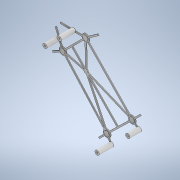
# Autodesk Inventor part: Grundform_Boden
Saved by Autodesk Inventor 2020.2 (Build 242310000, 310)
## iProperties
Created: 2020-03-04
Part Number: Grundform_Boden
Material: Generic
Document SubType Name: Modeling
Designer: Mara
Density: 1 g/cm^3
Appearance: Default
Author: Mara
Autodesk Inventor part; units mm, degrees
ref_plane "YZ Plane" through (0, 0, 0) normal (1, 0, 0) x (0, 1, 0)
ref_plane "XZ Plane" through (0, 0, 0) normal (0, 1, 0) x (-1, 0, 0)
ref_plane "XY Plane" through (0, 0, 0) normal (0, 0, 1) x (1, 0, 0)
sketch "Sketch1" plane through (0, 0, 0) normal (0, 0, 1) x (1, 0, 0)
  line L0 (-49.2977, 34.5359) -> (-22.38, 61.3045)
  line L1 (-47.8874, 33.1177) -> (-20.9698, 59.8864)
  line L2 (-49.2977, 34.5359) -> (-47.8874, 33.1177) construction
  circle A0 centre (-52.4729, 29.968) radius 5.563
  circle A1 centre (-52.4729, 29.968) radius 3.9984
  circle A2 centre (-17.7815, 64.4351) radius 5.563
  circle A3 centre (-17.7815, 64.4351) radius 3.9984
  line L3 (-13.9364, 68.4553) -> (0.7038, 78.9274)
  line L4 (-12.7631, 66.8356) -> (1.8771, 77.3077)
  line L5 (-57.711, 28.0946) -> (-68.2683, 22.3899)
  line L6 (-56.7093, 26.3625) -> (-67.2666, 20.6578)
  line L7 (-49.5894, 25.2106) -> (10.1162, -41.4966)
  circle A4 centre (14.4958, -44.9268) radius 5.563
  circle A5 centre (14.4958, -44.9268) radius 3.9984
  circle A6 centre (52.6405, -7.8239) radius 3.9984
  circle A7 centre (52.6405, -7.8239) radius 5.563
  line L8 (-48.0932, 26.5378) -> (11.6124, -40.1694)
  line L9 (-14.6001, 59.8716) -> (48.0505, -4.6808)
  line L10 (-13.1915, 61.292) -> (49.4591, -3.2604)
  line L11 (49.4227, -12.3618) -> (19.1106, -41.8201)
  line L12 (48.0258, -10.9306) -> (17.7136, -40.3888)
  line L13 (11.2885, -49.4721) -> (3.1929, -57.3557)
  line L14 (9.8883, -48.0441) -> (1.7927, -55.9277)
  line L15 (57.2511, -4.7111) -> (65.8331, 3.6764)
  line L16 (55.8523, -3.2817) -> (64.4343, 5.1058)
  line L17 (-39.0119, 41.9442) -> (29.6903, -28.7495)
  line L18 (-37.5936, 43.3546) -> (31.1246, -27.3556)
  line L19 (-55.5021, 34.6339) -> (-63.8979, 55.9393)
  line L20 (-53.6558, 35.4038) -> (-62.0516, 56.7092)
  line L21 (-23.223, 65.5915) -> (-56.073, 66.1322)
  line L22 (-23.2803, 63.5921) -> (-56.1303, 64.1329)
  circle A8 centre (-17.2221, 20.9576) radius 3.1804
  line L23 (13.0651, -39.5509) -> (-14.9644, 18.7175)
  line L24 (11.2563, -40.4044) -> (-16.7485, 17.8127)
  line L25 (-14.0533, 20.686) -> (47.9022, -4.9092)
  line L26 (-14.8421, 18.848) -> (47.1775, -6.7738)
  line L27 (-18.703, 58.9489) -> (-18.2564, 23.9652)
  line L28 (-16.7032, 58.9776) -> (-16.2565, 23.9879)
  line L29 (-47.4654, 27.5447) -> (-20.389, 20.6653)
  line L30 (-46.932, 29.4728) -> (-19.9371, 22.614)
  line L31 (0.7038, 78.9274) -> (1.8771, 77.3077)
  line L32 (-56.073, 66.1322) -> (-56.1303, 64.1329)
  line L33 (-62.0516, 56.7092) -> (-63.8979, 55.9393)
  line L34 (-68.2683, 22.3899) -> (-67.2666, 20.6578)
  line L35 (3.1929, -57.3557) -> (1.7927, -55.9277)
  line L36 (65.8331, 3.6764) -> (64.4343, 5.1058)
  point P0 (0, 0)
  point P1 (9.143, -43.4122)
  point P2 (-19.963, 60.8956)
  point P3 (18.6755, -41.2556)
  point P4 (19.8991, -43.603)
  point P5 (47.2964, -9.3692)
  point P6 (58.0343, -9.1855)
  point P7 (55.8444, -3.2761)
  point P8 (16.2732, -50.1982)
  point P9 (18.0227, -49.2289)
  point P10 (56.2951, -12.0181)
  point P11 (57.5423, -10.4544)
  point P12 (-20.321, 22.7115)
  point P13 (-20.9757, 59.8805)
  point P14 (-18.6091, 23.8197)
  point P15 (10.5981, -39.0362)
  point P16 (31.0842, -30.1838)
  point P17 (32.5185, -28.7899)
  point P18 (31.1246, -27.3556)
  point P19 (-13.0632, 18.1131)
  point P20 (-13.5186, 15.7119)
  point P21 (29.6903, -28.7495)
  point P22 (-20.0433, 22.4258)
  dimension "d49" = 6.3609
  dimension "d0" = 2
  dimension "d2" = 1
  dimension "d3" = 5.563
  dimension "d4" = 1.5646
  dimension "d6" = 1.5646
  dimension "d8" = 5.563
  dimension "d9" = 2
  dimension "d10" = 170.735
  dimension "d11" = 2
  dimension "d12" = 163.544
  dimension "d13" = 1.5646
  dimension "d17" = 7.9968
  dimension "d18" = 1.5646
  dimension "d19" = 7.9968
  dimension "d21" = 60.4275
  dimension "d22" = 66.8436
  dimension "d24" = 47.2075
  dimension "d25" = 2
  dimension "d26" = 2
  dimension "d27" = 81.433
  dimension "d28" = 93.011
  dimension "d29" = 53.2188
  dimension "d30" = 2
  dimension "d31" = 2
  dimension "d32" = 2
  dimension "d33" = 2
  dimension "d34" = 2
  dimension "d35" = 2
  dimension "d36" = 66.667
  dimension "d37" = 45.784
  dimension "d39" = 92.41
  dimension "d40" = 87.648
  dimension "d42" = 89.8
  dimension "d45" = 1
  dimension "d46" = 18
  dimension "d48" = 2
  dimension "d50" = 53.2132
  dimension "d51" = 27.126
  dimension "d52" = 44.9268
  dimension "d53" = 48.9027
  dimension "d54" = 29.968
  dimension "d55" = 20.9576
  dimension "d56" = 2
  dimension "d57" = 2
  dimension "d58" = 2
  dimension "d59" = 64.6596
  dimension "d60" = 67.0343
  dimension "d61" = 34.9897
  dimension "d62" = 27.8525
  dimension "d63" = 22.9
  dimension "d64" = 12
  dimension "d65" = 32.85
  dimension "d66" = 18
  dimension "d67" = 12
  dimension "d70" = 11.3
  dimension "d71" = 3.8451
  dimension "d72" = 5.4415
  dimension "d73" = 5.4358
  dimension "d74" = 5.2381
  dimension "d75" = 5.5409
  dimension "d76" = 5.4575
  dimension "d77" = 3.1128
  dimension "d78" = 2.6305
  dimension "d79" = 4.3021
  constraints: 75 end point, 25 parallel, 4 centre point, 4 coincident, 4 point on line, 2 perpendicular, 62 other
  measures "d0" distance between parallel lines of L1 L0
  measures "d2" distance from line of L0 point (-52.473, 29.968)
  measures "d3" distance of L0.start point (-52.473, 29.968)
  measures "d8" distance of L0.end point (-17.782, 64.435)
  measures "d9" distance between parallel lines of L4 L3
  measures "d10" angle of L3 L0
  measures "d11" distance between parallel lines of L6 L5
  measures "d12" angle of L1 L6
  measures "d17" diameter of A5
  measures "d19" diameter of A6
  measures "d21" distance of point (-52.473, 29.968) point (0, 0)
  measures "d22" distance of point (0, 0) point (-17.782, 64.435)
  measures "d24" distance of point (0, 0) point (14.496, -44.927)
  measures "d25" distance between parallel lines of L7 L8
  measures "d26" distance between parallel lines of L9 L10
  measures "d27" angle of L10 L4
  measures "d28" angle of L8 L1
  measures "d29" distance of point (0, 0) point (52.641, -7.824)
  measures "d30" distance between parallel lines of L11 L12
  measures "d31" distance between parallel lines of L13 L14
  measures "d32" distance between parallel lines of L15 L16
  measures "d33" distance between parallel lines of L18 L17
  measures "d34" distance between parallel lines of L20 L19
  measures "d35" distance between parallel lines of L21 L22
  measures "d36" angle of L0 L20
  measures "d37" angle of L0 L22
  measures "d39" angle of L14 L7
  measures "d40" angle of L12 L8
  measures "d42" angle of L10 L16
  measures "d45" distance from line of point (-17.222, 20.958) L18
  measures "d46" distance from line of L17 point (-52.473, 29.968)
  measures "d48" distance between parallel lines of L23 L24
  measures "d50" distance of point (52.641, -7.824) A5.centre
  measures "d51" distance of point (0, 0) point (-17.222, 20.958)
  measures "d52" vertical distance of point (0, 0) point (14.496, -44.927)
  measures "d53" distance of point (-52.473, 29.968) point (-17.782, 64.435)
  measures "d54" vertical distance of point (0, 0) point (-52.473, 29.968)
  measures "d55" vertical distance of point (-17.222, 20.958) point (0, 0)
  measures "d56" distance between parallel lines of L26 L25
  measures "d57" distance between parallel lines of L28 L27
  measures "d58" distance between parallel lines of L29 L30
  measures "d59" distance of L23.start L23.end
  measures "d60" distance of L25.start L25.end
  measures "d61" vertical distance of L28.start L28.end
  measures "d62" distance of L30.start L30.end
  measures "d63" distance of L20.start L20.end
  measures "d64" distance of L5.start L5.end
  measures "d65" horizontal distance of L22.start L22.end
  measures "d66" distance of L3.start L3.end
  measures "d67" distance of L15.start L15.end
  measures "d70" distance of L13.start L13.end
  measures "d71" horizontal distance of L3.start point (-17.782, 64.435)
  measures "d72" horizontal distance of point (-17.782, 64.435) L21.start
  measures "d73" vertical distance of point (-52.473, 29.968) L20.start
  measures "d74" horizontal distance of L5.start A1.centre
  measures "d75" horizontal distance of point (-52.473, 29.968) L30.start
  measures "d76" vertical distance of point (-17.782, 64.435) L28.start
  measures "d77" vertical distance of point (52.641, -7.824) L15.start
  measures "d78" vertical distance of point (52.641, -7.824) point (57.542, -10.454)
  measures "d79" vertical distance of A5.centre point (18.023, -49.229)
extrude "Extrusion3" add sketch "Sketch1" against normal blind 1 contours L0 A2 L1 A0 | A0 | A2 | A0 L19 L33 L20 | L22 L32 L21 A2 | L1 L18 A8 L30 L17 | A2 L28 A8 L27 | L17 A8 L29 A0 L30 | A0 L6 L34 L5 | L3 L31 L4 A2 | A8 L18 | L18 A8 L17 | L17 A8 | A8 L25 A7 L26 L18 | L18 L26 A8 | A2 L10 A7 L9 | A8 L23 L17 | L17 L23 A4 L8 L24 A8 | L8 L24 A4 L7 A0 | L18 L12 L17 L23 A8 L26 | A7 | L8 A4 L24 | A4 | L12 A7 L11 A4 | A4 L13 L35 L14 | L16 L36 L15 A7
sketch "Sketch3" plane through (0, 0, 0) normal (0, 0, 1) x (1, 0, 0)
  circle A0 centre (20.7546, -56.5669) radius 2.3783
  circle A1 centre (20.7546, -56.5669) radius 3.3783
  circle A2 centre (-36.8834, 64.7402) radius 2.3783
  circle A3 centre (-36.8834, 64.7402) radius 3.3783
  circle A4 centre (-58.3828, 44.2123) radius 2.3783
  circle A5 centre (-58.3828, 44.2123) radius 3.3783
  arc A6 (49.4227, -12.3618) -> (57.2511, -4.7111) centre (52.6405, -7.8239) ccw projected
  arc A7 (11.2885, -49.4721) -> (19.1106, -41.8201) centre (14.4958, -44.9268) ccw projected
  point P0 (0, 0)
  dimension "d93" = 1
  dimension "d94" = 4.7566
  dimension "d95" = 1
  dimension "d96" = 4.7566
  dimension "d99" = 1
  dimension "d100" = 4.7566
  constraints: 6 centre point, 3 coincident
  measures "d93" radial gap between concentric circles of A1 A0
  measures "d94" diameter of A0
  measures "d95" radial gap between concentric circles of A3 A2
  measures "d96" diameter of A2
  measures "d99" radial gap between concentric circles of A5 A4
  measures "d100" diameter of A4
sketch "Sketch5" plane through (0, 0, -1) normal (0, 0, -1) x (-1, 0, 0)
  circle A0 centre (-52.6405, -7.8239) radius 3.9984
  circle A1 centre (-52.6405, -7.8239) radius 3.9984 projected
  circle A2 centre (-14.4958, -44.9268) radius 3.9984
  circle A3 centre (-14.4958, -44.9268) radius 3.9984 projected
  circle A4 centre (52.4729, 29.968) radius 3.9984
  circle A5 centre (52.4729, 29.968) radius 3.9984 projected
  circle A6 centre (17.7815, 64.4351) radius 3.9984
  circle A7 centre (17.7815, 64.4351) radius 3.9984 projected
  point P0 (0, 0)
  constraints: 4 centre point, 4 coincident, 4 concentric
extrude "Extrusion4" add sketch "Sketch5" against normal blind 1.5
extrude "Extrusion5" add sketch "Sketch3" along normal blind 21 and the other way blind 1
sketch "Sketch6" plane through (0, 0, 0) normal (0, 0, 1) x (1, 0, 0)
  circle A0 centre (62.8402, -15.6905) radius 2.3785
  circle A1 centre (62.8402, -15.6905) radius 3.3785
  point P0 (0, 0)
  dimension "d109" = 4.757
  dimension "d110" = 1
  constraints: 2 centre point, 1 coincident
  measures "d109" diameter of A0
  measures "d110" radial gap between concentric circles of A1 A0
extrude "Extrusion6" add sketch "Sketch6" along normal blind 16.5 and the other way blind 1
sketch "Sketch7" plane through (-58.3828, 44.2123, 21) normal (0, 0, 1) x (1, 0, 0)
  circle A0 centre (0, 0) radius 3.3783
  circle A1 centre (0, 0) radius 3.3783 projected
  circle A2 centre (0, 0) radius 1.3297
  circle A3 centre (21.4994, 20.5278) radius 3.3783
  circle A4 centre (21.4994, 20.5278) radius 3.3783 projected
  circle A5 centre (21.4994, 20.5278) radius 1.3293
  circle A6 centre (79.1375, -100.7793) radius 3.3783
  circle A7 centre (79.1375, -100.7793) radius 3.3783 projected
  circle A8 centre (79.1375, -100.7793) radius 1.3293
  point P0 (58.3828, -44.2123)
  dimension "d115" = 2.0486
  dimension "d116" = 2.049
  dimension "d117" = 2.049
  constraints: 6 centre point, 6 coincident, 3 concentric
  measures "d115" radial gap between concentric circles of A0 A2
  measures "d116" radial gap between concentric circles of A3 A5
  measures "d117" radial gap between concentric circles of A6 A8
extrude "Extrusion7" add sketch "Sketch7" against normal blind 1
sketch "Sketch8" plane through (62.8402, -15.6905, 16.5) normal (0, 0, 1) x (1, 0, 0)
  circle A0 centre (0, 0) radius 3.3785
  circle A1 centre (0, 0) radius 3.3785 projected
  circle A2 centre (0, 0) radius 1.3295
  point P0 (-62.8402, 15.6905)
  dimension "d120" = 2.049
  constraints: 2 centre point, 2 coincident, 1 concentric
  measures "d120" radial gap between concentric circles of A0 A2
extrude "Extrusion8" add sketch "Sketch8" against normal blind 1
sketch "Sketch9" plane through (0, 0, -1) normal (0, 0, -1) x (-1, 0, 0)
  circle A0 centre (58.3828, 44.2123) radius 2.3783
  arc A1 (58.0553, 46.568) -> (56.5363, 42.7134) centre (58.3828, 44.2123) ccw projected
  circle A2 centre (36.8834, 64.7402) radius 2.3783
  arc A3 (34.7075, 63.7802) -> (39.0899, 63.8524) centre (36.8834, 64.7402) ccw projected
  point P0 (0, 0)
  constraints: 2 centre point, 2 coincident, 2 concentric
extrude "Extrusion9" cut sketch "Sketch9" against normal blind 2
sketch "Sketch10" plane through (0, 0, 0) normal (0, 0, 1) x (1, 0, 0)
  arc A0 (49.4227, -12.3618) -> (57.2511, -4.7111) centre (52.6405, -7.8239) ccw projected
  line L0 (56.3201, -11.9961) -> (59.655, -14.5641)
  circle A1 centre (62.8402, -15.6905) radius 3.3785 projected
  line L1 (57.5579, -10.4251) -> (60.8502, -12.9602)
  arc A2 (11.2885, -49.4721) -> (19.1106, -41.8201) centre (14.4958, -44.9268) ccw projected
  line L2 (16.2829, -50.1949) -> (18.3621, -54.1818)
  circle A3 centre (20.7546, -56.5669) radius 3.3783 projected
  line L3 (18.0312, -49.2219) -> (20.1301, -53.2468)
  circle A4 centre (20.7546, -56.5669) radius 3.3783 projected
  arc A5 (11.2885, -49.4721) -> (19.1106, -41.8201) centre (14.4958, -44.9268) ccw projected
  point P0 (0, 0)
  dimension "d125" = 2
  dimension "d127" = 2
  constraints: 8 end point, 7 point on circle, 2 parallel, 2 other
  measures "d125" distance between parallel lines of L1 L0
  measures "d127" distance between parallel lines of L2 L3
extrude "Extrusion10" add sketch "Sketch10" against normal blind 1 contours A0 L1 A1 L0 | A2 L3 A3 L2
equation "\"d6\" = d4"
equation "\"d8\" = d3"
equation "\"d13\" = d15"
equation "\"d18\" = d20"
equation "\"d15\" = 1.564594"
equation "\"d20\" = 1.564594"
body "Solid1"
